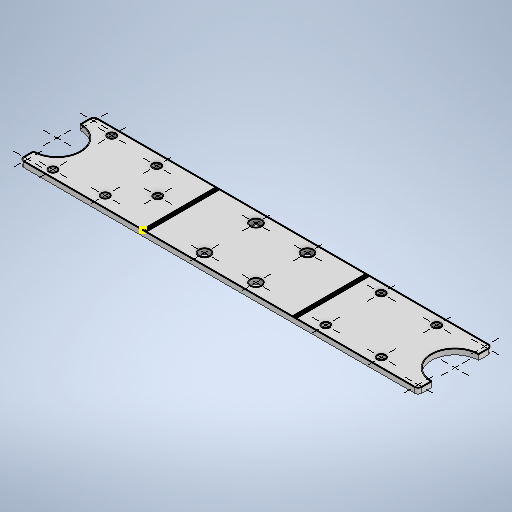
# Autodesk Inventor part: CAM_axis_5_top_frame
Saved by Autodesk Inventor 2025.2 (Build 292293000, 293)
## iProperties
Created: 2025-08-09
Part Number: CAM_axis_5_top_frame
Material: Generic
Document SubType Name: Modeling
Designer: User
Density: 1 g/cm^3
Appearance: Default
Author: User
Autodesk Inventor part; units mm, degrees
ref_plane "YZ Plane" through (0, 0, 0) normal (1, 0, 0) x (0, 1, 0)
ref_plane "XZ Plane" through (0, 0, 0) normal (0, 1, 0) x (-1, 0, 0)
ref_plane "XY Plane" through (0, 0, 0) normal (0, 0, 1) x (1, 0, 0)
sketch "Sketch1" plane through (0, 0, 0) normal (0, 1, 0) x (-1, 0, 0)
  line L0 (-0.4496, -20) -> (-0.4496, 0)
  line L1 (-41.2289, 0) -> (-41.2289, -20)
  circle A0 centre (13.17, -3) radius 1.05
  circle A1 centre (5.87, -10) radius 1.05
  circle A2 centre (13.17, -17) radius 1.05
  circle A3 centre (26.39, -18) radius 1.05
  circle A4 centre (26.39, -2) radius 1.05
  circle A5 centre (-62.4686, -2.475) radius 1.05
  circle A6 centre (-62.4686, -17.525) radius 1.05
  circle A7 centre (-47.3686, -17.525) radius 1.05
  circle A8 centre (-47.3686, -2.475) radius 1.05
  circle A9 centre (-13.8393, -17) radius 1.5
  circle A10 centre (-13.8393, -3) radius 1.5
  circle A11 centre (-27.8393, -3) radius 1.5
  circle A12 centre (-27.8393, -17) radius 1.5
  arc A13 (32.29, -20) -> (33.29, -19) centre (32.29, -19) ccw
  line L2 (33.29, -19) -> (33.29, -16.4)
  arc A14 (33.29, -1) -> (32.29, 0) centre (32.29, -1) ccw
  line L3 (33.29, -3.6) -> (33.29, -1)
  arc A15 (-73.9686, 0) -> (-74.9686, -1) centre (-73.9686, -1) ccw
  arc A16 (-74.9686, -19) -> (-73.9686, -20) centre (-73.9686, -19) ccw
  line L4 (-74.9686, -1) -> (-74.9686, -3.6)
  line L5 (-74.9686, -16.4) -> (-74.9686, -19)
  arc A17 (33.29, -3.6) -> (33.29, -16.4) centre (33.29, -10) ccw
  arc A18 (-74.9686, -16.4) -> (-74.9686, -3.6) centre (-74.9686, -10) ccw
  line L6 (32.29, -20) -> (-73.9686, -20)
  line L7 (-73.9686, 0) -> (32.29, 0)
  line L8 (-41.6786, -20) -> (-41.6786, 0)
  line L9 (-40.7793, 0) -> (-40.7793, -20)
  line L10 (-0.8993, -20) -> (-0.8993, 0)
  line L11 (0, 0) -> (0, -20)
  constraints: 24 end point, 19 centre point, 15 equal radius, 12 point on circle, 12 point on line, 11 tangent, 10 vertical, 8 parallel, 2 horizontal, 2 perpendicular, 63 other
extrude "Extrusion1" add sketch "Sketch1" against normal blind 1.5
body "Solid1"
